Autodesk Inventor part; units mm, degrees
(part 2 of 2)
extrude "押し出し10" add sketch "スケッチ5" against normal blind 1 contours L272 A37 L310 L314 L315 L296 L297 L277 L300 L299 L318 L317 L322 L274 A39 L233 L235 L234 L284 L285 L238 L292 L291 L290 L283 L282 L231 L232 L230 | L272 A36 A37 | L272 A36 | L272 L248 L260 L314 L310 | L272 L308 L275 L258 | L272 L258 L275 L313 L314 L260 L248 | L314 L260 L275 L310 | L310 L275 L295 L315 L314 | L272 L273 L265 L267 L268 L269 L294 L274 L320 L276 L293 L270 L271 L275 L308 | L314 L313 L275 L260 | L290 L291 L292 L238 | L277 L297 L296 L295 | L265 L269 L268 L267 | L277 L298 L299 L300 | L276 L322 L317 L318 L298 | L276 L263 L317 L322 | L320 L274 L261 L276 | L276 L316 L317 L263 | L317 L263 L262 L274 L322 | L261 L274 L262 L263 L317 L316 L276 | L274 A38 A39 | L274 A38 | L301 L302 L303 L278 | L306 L305 L304 L278 | A19 | A20 | A22 | A23 | A25 | A26 | A28 | A29 | A30 | A33 | L326 L327 L328 L329 | L335 L334 L333 L332 | A41 | A42 picked at (-27.253467, 18.674544) picked at (-28.499793, 18.668966) picked at (27.276729, 18.207249) picked at (28.427979, 18.259216)
extrude "押し出し11" cut sketch "スケッチ5" against normal blind 1.5 contours L277 L297 L296 L295 | L277 L298 L299 L300 | L301 L302 L303 L278 | L306 L305 L304 L278
chamfer "面取り8" distance 2 angle 45 2 edges at (-24.8255, 13.5, -0.5) (24.8255, 13.5, -0.5)
chamfer "面取り9" distance 1 angle 45 2 edges at (-24.2643, -13.5, -0.5) (24.2643, -13.5, -0.5)
extrude "押し出し12" add sketch "スケッチ5" against normal blind 1 contours L286 L287 L311 L310 L272 A37 | A37 L272 A36 | A36 L272 | L287 L272 L258 L248 L310 L311 | L248 L258 L272 | L322 L323 L289 L288 L274 A39 | L274 L262 L261 L289 L323 L322 | L261 L262 L274 | A39 L274 A38 | A38 L274 picked at (-29.723249, 18.793105) picked at (-29.04927, 18.620878) picked at (29.202957, 17.455508) picked at (29.040228, 18.534292)
chamfer "面取り10" distance 2 angle 45 2 edges at (-31, 8.5, -0.5) (31, 8.5, -0.5)
chamfer "面取り11" distance 0.8 angle 45 2 edges at (-31, -8.5, -0.5) (31, -8.5, -0.5)
extrude "押し出し13" cut sketch "スケッチ5" against normal blind 1.5 contours A19 | A22 | A25 | A28
extrude "押し出し14" cut sketch "スケッチ5" against normal blind 1.5 contours A30 | A33
extrude "押し出し15" cut sketch "スケッチ5" against normal blind 1.5 contours L314 L260 L275 L310 | L310 L275 L295 L315 L314 | L314 L313 L275 L260 | L277 L297 L296 L295
chamfer "面取り12" distance 2 angle 45 1 edges at (-26, 13.5, -0.5)
extrude "押し出し16" cut sketch "スケッチ5" against normal blind 1.5 contours L277 L298 L299 L300 | L276 L322 L317 L318 L298 | L276 L263 L317 L322 | L276 L316 L317 L263
chamfer "面取り13" distance 2 angle 45 1 edges at (26, 13.5, -0.5)
extrude "押し出し17" cut sketch "スケッチ5" against normal blind 1.5 contours A36 L272 | L272 A36
extrude "押し出し18" cut sketch "スケッチ5" against normal blind 1.5 contours A38 L274 | L274 A38
extrude "押し出し19" cut sketch "スケッチ5" against normal blind 1.5 contours L265 L269 L268 L267
extrude "押し出し20" cut sketch "スケッチ5" against normal blind 1.5 contours L290 L291 L292 L238
fillet "フィレット1" radius 0.8 4 edges at (-19, 8.5, -0.5) (-19, -8.5, -0.5) (19, -8.5, -0.5) (19, 8.5, -0.5)
fillet "フィレット2" radius 0.8 26 edges at (-26, 15.5, -0.5) (-24, 13.5, -0.5) (-20.8255, 13.5, -0.5) (-15.3255, 19, -0.5) (15.3255, 19, -0.5) (20.8255, 13.5, -0.5) (24, 13.5, -0.5) (26, 15.5, -0.5) (26, 24.1685, -0.5) (21.8107, 27.6837, -0.5) (-26, 24.1685, -0.5) (-21.8107, 27.6837, -0.5) (-18.1736, 44.795, -0.5) (-8.7095, 51.4218, -0.5) (8.7095, 51.4218, -0.5) (18.1736, 44.795, -0.5) (-23.55, -14.1999, -0.5) (-23.2643, -13.5, -0.5) (-21.2643, -13.5, -0.5) (-11.6308, -20, -0.5) (-11.5077, -26, -0.5) (11.5077, -26, -0.5) (11.6308, -20, -0.5) (21.2643, -13.5, -0.5) (23.55, -14.1999, -0.5) (23.2643, -13.5, -0.5)
fillet "フィレット3" radius 0.8 28 edges at (-6.6203, -29.5, -0.5) (-8.1203, -31, -0.5) (-12.1203, -31, -0.5) (6.6203, -29.5, -0.5) (8.1203, -31, -0.5) (12.1203, -31, -0.5) (31, -12.5, -0.5) (31, -9.3, -0.5) (30.2, -8.5, -0.5) (29, 8.5, -0.5) (31, 10.5, -0.5) (31, 26.5, -0.5) (26.3435, 30.4073, -0.5) (22.0451, 50.6295, -0.5) (13.7728, 56.4218, -0.5) (7.7728, 56.4218, -0.5) (5.0254, 55.4218, -0.5) (-5.0254, 55.4218, -0.5) (-7.7728, 56.4218, -0.5) (-13.7728, 56.4218, -0.5) (-22.0451, 50.6295, -0.5) (-26.3435, 30.4073, -0.5) (-31, 26.5, -0.5) (-31, 10.5, -0.5) (-29, 8.5, -0.5) (-30.2, -8.5, -0.5) (-31, -9.3, -0.5) (-31, -12.5, -0.5)
extrude "押し出し21" cut sketch "スケッチ5" against normal blind 2 contours L326 L327 L328 L329 | L335 L334 L333 L332 | A41 | A42
